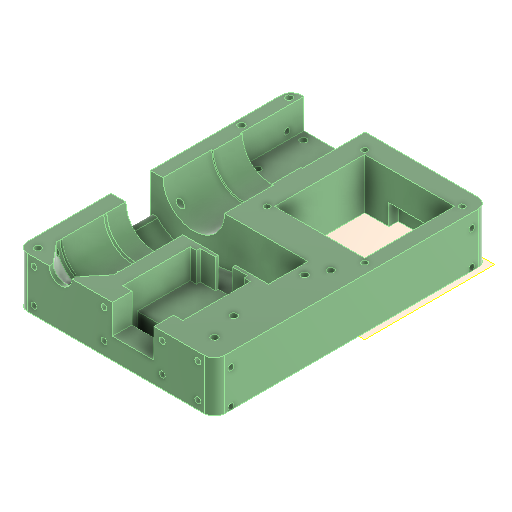
# Autodesk Inventor part: 60_Planktoscope_Base_half1
Saved by Autodesk Inventor 2024.1 (Build 281209000, 209)
## iProperties
Created: 2024-03-03
Part Number: 60_Planktoscope_Base_half1
Material: Generisch
Document SubType Name: Modeling
Designer: diederichbenedict
Density: 1 g/cm^3
Appearance: Glatt - Waldgrün
Author: diederichbenedict
Autodesk Inventor part; units mm, degrees
ref_plane "YZ Plane" through (0, 0, 0) normal (1, 0, 0) x (0, 1, 0)
ref_plane "XZ Plane" through (0, 0, 0) normal (0, 1, 0) x (-1, 0, 0)
ref_plane "Arbeitsebene1" through (0, 0, 0) normal (0, 0, 1) x (1, 0, 0)
ref_plane "Arbeitsebene2" through (-59.4, -108.46, 24.3) normal (0, 0, -1) x (0, 1, 0)
sketch "Skizze1" plane through (0, 0, 0) normal (0, 0, 1) x (1, 0, 0)
  line L0 (-24.5, 28.5) -> (24.5, 28.5) construction
  arc A0 (-24.5, 28.5) -> (-28.5, 24.5) centre (-24.5, 24.5) ccw construction
  line L1 (-28.5, -24.5) -> (-28.5, 24.5) construction
  arc A1 (-28.5, -24.5) -> (-24.5, -28.5) centre (-24.5, -24.5) ccw construction
  line L2 (24.5, -28.5) -> (-24.5, -28.5) construction
  arc A2 (24.5, -28.5) -> (28.5, -24.5) centre (24.5, -24.5) ccw construction
  line L3 (28.5, 24.5) -> (28.5, -24.5) construction
  arc A3 (28.5, 24.5) -> (24.5, 28.5) centre (24.5, 24.5) ccw construction
  circle A4 centre (15.5, -15.5) radius 2 construction
  circle A5 centre (-15.5, -15.5) radius 2 construction
  circle A6 centre (-15.5, 15.5) radius 2 construction
  circle A7 centre (15.5, 15.5) radius 2 construction
  circle A8 centre (0, 0) radius 11.5 construction
  circle A9 centre (23.5, -23.5) radius 2 construction
  circle A10 centre (-23.5, -23.5) radius 2 construction
  circle A11 centre (-23.5, 23.5) radius 2 construction
  circle A12 centre (23.5, 23.5) radius 2 construction
  line L4 (21.15, 14.15) -> (21.15, -14.15) construction
  line L5 (14.15, 21.15) -> (21.15, 14.15) construction
  line L6 (-14.15, 21.15) -> (14.15, 21.15) construction
  line L7 (-21.15, 14.15) -> (-14.15, 21.15) construction
  line L8 (-21.15, -14.15) -> (-21.15, 14.15) construction
  line L9 (-14.15, -21.15) -> (-21.15, -14.15) construction
  line L10 (14.15, -21.15) -> (-14.15, -21.15) construction
  line L11 (21.15, -14.15) -> (14.15, -21.15) construction
  line L12 (17.15, 21.15) -> (14.15, 21.15) construction
  line L13 (21.15, 14.15) -> (14.15, 21.15) construction
  line L14 (21.15, 14.15) -> (21.15, 17.15) construction
  line L15 (21.15, 17.15) -> (17.15, 21.15) construction
  line L16 (21.1433, 21.15) -> (-21.15, 21.15) construction
  line L17 (-21.15, 21.15) -> (-21.15, -21.15) construction
  line L18 (-21.15, -21.15) -> (21.1433, -21.15) construction
  line L19 (21.1433, -21.15) -> (21.1433, 21.15) construction
  line L20 (21.6433, 21.65) -> (-21.65, 21.65)
  line L21 (-21.65, 21.65) -> (-21.65, -21.65)
  line L22 (-21.65, -21.65) -> (21.6433, -21.65)
  line L23 (21.6433, -21.65) -> (21.6433, 21.65)
  circle A13 centre (23.5, 23.5) radius 1.4
  circle A14 centre (23.5, -23.5) radius 1.4
  circle A15 centre (-23.5, 23.5) radius 1.4
  circle A16 centre (-23.5, -23.5) radius 1.4
  line L24 (-58.0629, 31.15) -> (-46.7147, 31.15) construction
  line L25 (-24.5, 28.5) -> (24.5, 28.5) construction
  line L26 (-58.15, -108.944) -> (-33.15, -108.944) construction
  line L27 (-60.15, 4.6456) -> (-60.15, 29.65) construction
  line L28 (28.5, 31.15) -> (-66.5, 31.15) construction
  line L29 (-66.5, 31.15) -> (-66.5, -100.85) construction
  line L30 (-66.5, -100.85) -> (28.5, -100.85) construction
  line L31 (28.5, -100.85) -> (28.5, 31.15) construction
  line L32 (28.5, 31.15) -> (-66.5, 31.15)
  line L33 (-66.5, 31.15) -> (-66.5, -100.85)
  line L34 (-66.5, -100.85) -> (28.5, -100.85)
  line L35 (28.5, -100.85) -> (28.5, 31.15)
  circle A17 centre (-34.65, 27.15) radius 1.6 projected
  circle A18 centre (-35.65, 4.15) radius 1.55 projected
  arc A19 (-35.0696, 29.65) -> (-37.5716, 27.1718) centre (-35.0717, 27.15) ccw construction
  line L36 (-32.3578, 29.6503) -> (-35.0696, 29.6501) construction
  line L37 (-32.3578, 29.6503) -> (-32.3574, 2.149) construction
  spline S0 degree 3 poles (-33.2494, 1.4648) (-33.1945, 1.4704) (-33.1402, 1.4798) (-33.0852, 1.4932) (-33.0302, 1.5066) (-32.9745, 1.5241) (-32.9218, 1.5443) (-32.869, 1.5646) (-32.8192, 1.5877) (-32.7741, 1.6117) (-32.729, 1.6358) (-32.6887, 1.6608) (-32.6523, 1.6864) (-32.6158, 1.712) (-32.5833, 1.7382) (-32.5542, 1.7648) (-32.5251, 1.7914) (-32.4996, 1.8183) (-32.4775, 1.8453) (-32.4554, 1.8722) (-32.4367, 1.899) (-32.4213, 1.9255) (-32.4059, 1.952) (-32.3937, 1.978) (-32.3842, 2.0033) (-32.3747, 2.0286) (-32.3679, 2.0532) (-32.3636, 2.0778) (-32.3593, 2.1023) (-32.3574, 2.1268) (-32.3574, 2.149) knots 0 0 0 0 0.1 0.1 0.1 0.2 0.2 0.2 0.3 0.3 0.3 0.4 0.4 0.4 0.5 0.5 0.5 0.6 0.6 0.6 0.7 0.7 0.7 0.8 0.8 0.8 0.9 0.9 0.9 1 1 1 1 construction
  spline S1 degree 3 poles (-58.0506, 1.4648) (-57.9483, 1.4544) (-57.7309, 1.4485) (-57.3891, 1.4505) (-57.0142, 1.4499) (-56.6055, 1.45) (-56.1597, 1.45) (-55.6728, 1.45) (-55.1399, 1.45) (-54.5557, 1.45) (-53.9136, 1.45) (-53.2059, 1.45) (-52.4235, 1.45) (-51.5547, 1.45) (-50.5859, 1.45) (-49.498, 1.45) (-48.2725, 1.45) (-46.9373, 1.45) (-45.5731, 1.45) (-44.2623, 1.45) (-43.0442, 1.45) (-41.9119, 1.45) (-40.8595, 1.45) (-39.8813, 1.45) (-38.9722, 1.45) (-38.1274, 1.45) (-37.3425, 1.45) (-36.6135, 1.45) (-35.9369, 1.45) (-35.3097, 1.45) (-34.7295, 1.45) (-34.1949, 1.45) (-33.7068, 1.4499) (-33.3956, 1.4501) (-33.2494, 1.4648) knots 0 0 0 0 0.012454 0.026265 0.041356 0.057789 0.075708 0.095278 0.116688 0.140158 0.165945 0.194355 0.225757 0.26059 0.299437 0.342945 0.392182 0.44767 0.504448 0.55719 0.606219 0.651791 0.694148 0.733518 0.770107 0.804111 0.835704 0.865049 0.892289 0.917546 0.940917 0.962464 0.982201 1 1 1 1 construction
  spline S2 degree 3 poles (-58.9429, 2.1479) (-58.9428, 2.1323) (-58.9408, 2.1003) (-58.9319, 2.0518) (-58.9165, 2.0024) (-58.8947, 1.9528) (-58.866, 1.9029) (-58.8299, 1.8528) (-58.786, 1.8026) (-58.7333, 1.7522) (-58.6711, 1.7019) (-58.5978, 1.6519) (-58.512, 1.6028) (-58.4118, 1.556) (-58.2981, 1.5143) (-58.1761, 1.4822) (-58.092, 1.469) (-58.0506, 1.4648) knots 0.000644 0.000644 0.000644 0.000644 0.046478 0.094952 0.144249 0.194804 0.247064 0.301535 0.358802 0.419552 0.484614 0.554981 0.631878 0.716385 0.809647 0.906987 1 1 1 1 construction
  line L38 (-58.9426, 2.1485) -> (-58.9422, 29.6503) construction
  line L39 (-58.9422, 29.6503) -> (-56.2298, 29.6501) construction
  arc A20 (-53.7284, 27.1718) -> (-56.2298, 29.65) centre (-56.2283, 27.15) ccw construction
  line L40 (-53.7228, 26.5387) -> (-53.7284, 27.1718) construction
  arc A21 (-53.7228, 26.5387) -> (-52.4229, 25.25) centre (-52.4229, 26.55) ccw construction
  line L41 (-38.8771, 25.25) -> (-52.4229, 25.25) construction
  arc A22 (-38.8771, 25.25) -> (-37.5772, 26.5387) centre (-38.8771, 26.55) ccw construction
  line L42 (-37.5772, 26.5387) -> (-37.5716, 27.1718) construction
  circle A23 centre (-56.65, 27.15) radius 1.6 projected
  line L43 (-58.35, 24.2) -> (-35.55, 24.2) construction
  line L44 (-58.35, 8.8) -> (-58.35, 24.2) construction
  line L45 (-32.95, 8.8) -> (-58.35, 8.8) construction
  line L46 (-32.95, 21.2) -> (-32.95, 8.8) construction
  line L47 (-35.55, 24.2) -> (-32.95, 21.2) construction
  circle A24 centre (-55.65, 4.15) radius 1.55 projected
  circle A25 centre (-51.65, 5.65) radius 1.1 construction
  circle A26 centre (-39.65, 5.65) radius 1.1 construction
  circle A27 centre (-35.65, 4.15) radius 1.55 construction
  circle A28 centre (-34.65, 27.15) radius 1.6 construction
  point P0 (0, 0)
  dimension "d0" = 0.5
  dimension "d1" = 2.8
  dimension "d2" = 2.8
  dimension "d3" = 2.8
  dimension "d4" = 2.8
  dimension "d5" = 95
  dimension "d6" = 132
  dimension "d41" = 31.15
  constraints: 32 end point, 8 parallel, 4 centre point, 4 coincident, 4 perpendicular, 3 horizontal, 3 other
  measures "d0" distance between parallel lines of L19 L23
  measures "d1" diameter of A13
  measures "d2" diameter of A14
  measures "d3" diameter of A15
  measures "d4" diameter of A16
  measures "d5" distance of L30.end L29.end
  measures "d6" distance of L29.end L28.end
  measures "d41" distance from line of L28 point (0, 0)
extrude "Extrusion1" add sketch "Skizze1" along normal up to surface (24.3 mm away)
sketch "Skizze2" plane through (-66.5, 31.15, 24.3) normal (0, 0, 1) x (1, 0, 0)
  line L0 (44.85, -9.5) -> (88.1433, -9.5) projected
  line L1 (88.1433, -9.5) -> (88.1433, -52.8) projected
  line L2 (88.1433, -52.8) -> (44.85, -52.8) projected
  line L3 (44.85, -52.8) -> (44.85, -9.5) projected
  circle A0 centre (90, -7.65) radius 1.4 projected
  circle A1 centre (90, -54.65) radius 1.4 projected
  circle A2 centre (43, -7.65) radius 1.4 projected
  circle A3 centre (43, -54.65) radius 1.4 projected
  circle A4 centre (31.85, -4) radius 1.6 projected
  circle A5 centre (30.85, -27) radius 1.55 projected
  circle A6 centre (9.85, -4) radius 1.6 projected
  circle A7 centre (10.85, -27) radius 1.55 projected
  line L4 (95, 0) -> (0, 0) projected
  line L5 (0, 0) -> (0, -132) projected
  line L6 (0, -132) -> (95, -132) projected
  line L7 (95, -132) -> (95, 0) projected
  line L8 (7.35, -118.91) -> (7.35, -120.06)
  arc A8 (7.35, -118.91) -> (7.35, -117.91) centre (7.35, -118.41) ccw construction
  line L9 (7.35, -96.06) -> (7.35, -117.91) construction
  line L10 (7.35, -85.56) -> (7.35, -94.56)
  line L11 (6.25, -85.56) -> (35.45, -85.56) projected
  line L12 (6.25, -70.56) -> (6.25, -85.56)
  line L13 (6.25, -44.56) -> (6.25, -70.06)
  line L14 (6.9535, -41.86) -> (6.8517, -30.1979)
  line L15 (33.2, -30.2) -> (33.2, -41.66)
  line L16 (6.9, -41.86) -> (6.9, -44.56)
  line L17 (6.25, -44.56) -> (35.45, -44.56) projected
  line L18 (20.85, -132) -> (20.85, 0) construction
  line L19 (15.35, -128.06) -> (15.35, -132)
  line L20 (7.35, -96.06) -> (7.35, -94.56)
  line L21 (7.35, -85.56) -> (6.25, -85.56)
  line L22 (6.25, -70.56) -> (6.25, -70.06)
  line L23 (15.1, -132) -> (15.1, -128.1636)
  line L24 (7.1, -120.1636) -> (7.1, -118.41)
  arc A9 (7.1, -118.41) -> (7.1, -118.41) centre (7.35, -118.41) ccw
  line L25 (7.1, -118.41) -> (7.1, -96.0507)
  line L26 (7.1, -96.0507) -> (7.1, -94.56)
  line L27 (7.1, -94.56) -> (7.1, -85.81)
  line L28 (7.1, -85.81) -> (6, -85.81)
  line L29 (6, -85.81) -> (6, -70.56)
  line L30 (6, -70.56) -> (6, -70.06)
  line L31 (6, -70.06) -> (6, -44.31)
  line L32 (6, -44.31) -> (35.45, -44.31)
  line L33 (6.8, -44.31) -> (6.8, -30.064)
  line L34 (6.8, -30.064) -> (20.85, -30.064)
  line L35 (20.85, -30.064) -> (20.85, -132)
  line L36 (15.1, -132) -> (20.85, -132)
  line L37 (7.1, -97.4127) -> (7.2407, -96.0654)
  line L38 (7.2407, -96.0654) -> (7.1, -96.0507)
  circle A10 centre (7.1, -117.9136) radius 0.5
  line L39 (7.35, -120.06) -> (15.35, -129.594) construction
  line L40 (15.35, -130.03) -> (7.1, -120.198)
  line L41 (7.1, -120.198) -> (7.1, -120.1636)
  point P0 (66.5, -31.15)
  point P1 (20.85, -85.56)
  point P2 (20.85, -44.56)
  point P3 (20.85, -44.31)
  point P4 (7.1, -118.4136)
  point P5 (7.1, -117.4136)
  point P6 (15.1, -129.7321)
  point P7 (6.9, -44.31)
  dimension "d9" = 0.25
  dimension "d74" = 1
  dimension "d75" = 2.25
  constraints: 64 end point, 11 vertical, 7 point on line, 5 perpendicular, 4 point on circle, 3 centre point, 2 collinear, 1 horizontal, 1 midpoint, 1 parallel, 30 other
  measures "d9" distance between parallel lines of L9 L25
  measures "d74" diameter of A10
  measures "d75" distance of A10.centre L24.start
revolve "Umdrehung1" cut sketch "Skizze2" angle 360 about axis through (-45.65, -100.85, 24.3) along (0, 1, 0) contours L6 L19 L40 L41 L24 A9 A10 L25 L37 L38 L26 L27 L28 L29 L30 L31 L32 L16 L17 L13 L22 L12 L11 L35 | L11 L12 L22 L13 L17 L35 | L17 L16 L32 L35 | L32 L33 L34 L35 | A10 A9
sketch "Skizze3" plane through (-66.5, 31.15, 24.3) normal (0, 0, 1) x (1, 0, 0)
  line L0 (41.8499, -119.66) -> (41.8499, -113.96) projected
  line L1 (69.8499, -119.66) -> (69.8499, -113.96) projected
  line L2 (47.9499, -122.06) -> (63.7499, -122.06) projected
  line L3 (44.8499, -88.76) -> (66.8499, -88.76) projected
  line L4 (44.8499, -90.56) -> (44.8499, -88.76)
  line L5 (66.8499, -90.56) -> (66.8499, -88.76)
  line L6 (41.8499, -122.06) -> (69.8499, -122.06)
  line L7 (69.8499, -122.06) -> (69.8499, -90.56)
  line L8 (69.8499, -90.56) -> (41.8499, -90.56)
  line L9 (41.8499, -90.56) -> (41.8499, -122.06)
  line L10 (65.8499, -140.6578) -> (45.8499, -140.6578)
  line L11 (45.8499, -140.6578) -> (45.8499, -122.06)
  line L12 (45.8499, -122.06) -> (65.8499, -122.06)
  line L13 (65.8499, -122.06) -> (65.8499, -140.6578)
  line L14 (65.8499, -140.6578) -> (45.8499, -122.06) construction
  line L15 (45.8499, -140.6578) -> (65.8499, -122.06) construction
  line L16 (41.3499, -122.56) -> (70.3499, -122.56)
  line L17 (70.3499, -122.56) -> (70.3499, -90.06)
  line L18 (70.3499, -90.06) -> (41.3499, -90.06)
  line L19 (41.3499, -90.06) -> (41.3499, -122.56)
  line L20 (67.3499, -90.56) -> (67.3499, -88.26)
  line L21 (67.3499, -88.26) -> (44.3499, -88.26)
  line L22 (44.3499, -88.26) -> (44.3499, -90.56)
  line L23 (60.0306, -74.6503) -> (51.6692, -74.6503)
  line L24 (51.6692, -74.6503) -> (51.6692, -88.26)
  line L25 (51.6692, -88.26) -> (60.0306, -88.26)
  line L26 (60.0306, -88.26) -> (60.0306, -74.6503)
  line L27 (60.0306, -74.6503) -> (51.6692, -88.26) construction
  line L28 (51.6692, -74.6503) -> (60.0306, -88.26) construction
  point P0 (66.5, -31.15)
  point P1 (55.8499, -131.3589)
  point P2 (55.8499, -81.4552)
  point P3 (44.3499, -90.06)
  point P4 (45.8499, -122.56)
  point P5 (65.8499, -122.56)
  point P6 (67.3499, -90.06)
  dimension "d11" = 20
  dimension "d12" = 0.5
  dimension "d13" = 0.5
  constraints: 50 end point, 8 parallel, 4 midpoint, 4 perpendicular, 3 horizontal, 2 point on line, 2 vertical, 7 other
  measures "d11" distance of L11.end L12.end
  measures "d12" distance between parallel lines of L9 L19
  measures "d13" distance between parallel lines of L3 L21
extrude "Extrusion2" cut sketch "Skizze3" against normal blind 14.1
sketch "Skizze4" plane through (-60.5, -54.66, 24.3) normal (0, 1, 0) x (1, 0, 0)
  arc A0 (14.7163, 14.1976) -> (0.6736, 0.7871) centre (14.85, 0) ccw projected
  circle A1 centre (49.8499, -0.1) radius 2.3 projected
  circle A2 centre (14.85, 0) radius 14.1983
  circle A3 centre (49.8499, -0.1) radius 6
  circle A4 centre (14.85, 0) radius 25.1983
  circle A5 centre (49.8499, -0.1) radius 20
  line L0 (18.6637, 24.908) -> (52.8768, 19.6696)
  line L1 (49.8499, -0.1) -> (14.85, 0)
  point P0 (60.5, 24.3)
  point P1 (40.0482, -0.072)
  point P2 (29.8499, -0.0429)
  point P3 (35.666, -14.2003)
  point P4 (35.7468, 14.0811)
  dimension "d16" = 12
  dimension "d17" = 11
  dimension "d18" = 14
  constraints: 4 end point, 2 centre point, 2 coincident, 1 concentric, 8 other
  measures "d16" diameter of A3
extrude "Extrusion3" cut sketch "Skizze4" along normal blind 18 and the other way blind 1 contours A2 A0 | A5 A4 | A5 A4 L1 | L1 A4 A5 | A1 | A3 | A5 A4 | A4 L0 A5
sketch "Skizze5" plane through (-66.5, 31.15, 24.3) normal (0, 0, 1) x (1, 0, 0)
  line L0 (60.0306, -86.81) -> (60.0306, -88.26) projected
  line L1 (60.0306, -88.26) -> (67.3499, -88.26) projected
  line L2 (67.3499, -88.26) -> (67.3499, -90.06) projected
  line L3 (67.3499, -90.06) -> (70.3499, -90.06) projected
  line L4 (70.3499, -90.06) -> (70.3499, -122.56) projected
  line L5 (70.3499, -122.56) -> (65.8499, -122.56) projected
  line L6 (65.8499, -122.56) -> (65.8499, -132) projected
  line L7 (65.8499, -132) -> (95, -132) projected
  line L8 (95, -132) -> (95, 0) projected
  line L9 (95, 0) -> (0, 0) projected
  line L10 (26.35, -132) -> (45.8499, -132) projected
  line L11 (44.85, -9.5) -> (88.1433, -9.5) projected
  line L12 (88.1433, -9.5) -> (88.1433, -52.8) projected
  line L13 (88.1433, -52.8) -> (44.85, -52.8) projected
  line L14 (44.85, -52.8) -> (44.85, -9.5) projected
  circle A0 centre (90, -7.65) radius 1.4 projected
  circle A1 centre (90, -54.65) radius 1.4 projected
  circle A2 centre (43, -7.65) radius 1.4 projected
  circle A3 centre (43, -54.65) radius 1.4 projected
  circle A4 centre (31.85, -4) radius 1.6 projected
  circle A5 centre (30.85, -27) radius 1.55 projected
  circle A6 centre (9.85, -4) radius 1.6 projected
  circle A7 centre (10.85, -27) radius 1.55 projected
  line L15 (35.35, -1.5) -> (35.35, -27) projected
  line L16 (6.35, -26.9997) -> (6.35, -1.5) projected
  line L17 (35.35, -30.064) -> (6.35, -30.064)
  line L18 (6.35, -30.064) -> (6.35, 0)
  line L19 (6.35, 0) -> (35.35, 0)
  line L20 (35.35, 0) -> (35.35, -30.064)
  line L21 (35.65, -30.364) -> (6.05, -30.364)
  line L22 (6.05, -30.364) -> (6.05, 0.3)
  line L23 (6.05, 0.3) -> (35.65, 0.3)
  line L24 (35.65, 0.3) -> (35.65, -30.364)
  line L25 (45.8499, -132) -> (45.8499, -122.56) projected
  line L26 (45.8499, -122.56) -> (41.3499, -122.56) projected
  line L27 (41.3499, -122.56) -> (41.3499, -90.06) projected
  line L28 (41.3499, -90.06) -> (44.3499, -90.06) projected
  line L29 (44.3499, -90.06) -> (44.3499, -88.26) projected
  line L30 (44.3499, -88.26) -> (51.6692, -88.26) projected
  line L31 (51.6692, -88.26) -> (51.6692, -86.81) projected
  line L32 (0, -86.81) -> (0, -132) projected
  line L33 (51.6692, -86.81) -> (34.6, -86.81) projected
  line L34 (34.6, -86.81) -> (34.6, -96.0507) projected
  line L35 (34.6, -96.0507) -> (34.4593, -96.0654) projected
  line L36 (34.4593, -96.0654) -> (34.6, -97.4127) projected
  line L37 (34.6, -97.4127) -> (34.6, -117.4136) projected
  arc A8 (34.6, -117.4136) -> (34.6, -118.4136) centre (34.6, -117.9136) ccw projected
  line L38 (34.6, -118.4136) -> (34.6, -120.198) projected
  line L39 (34.6, -120.198) -> (26.35, -130.03) projected
  line L40 (26.35, -130.03) -> (26.35, -132) projected
  line L41 (75.8496, -86.81) -> (60.0306, -86.81) projected
  line L42 (0, 0) -> (0, -67.81) projected
  line L43 (0, -67.81) -> (6, -67.81) projected
  line L44 (6, -67.81) -> (6, -44.31) projected
  line L45 (6, -44.31) -> (6.8, -44.31) projected
  line L46 (6.8, -44.31) -> (6.8, -30.064) projected
  line L47 (6.8, -30.064) -> (34.9, -30.064) projected
  line L48 (34.9, -30.064) -> (34.9, -44.31) projected
  line L49 (34.9, -44.31) -> (35.7, -44.31) projected
  line L50 (35.7, -44.31) -> (35.7, -67.81) projected
  line L51 (35.7, -67.81) -> (75.8496, -67.81) projected
  line L52 (75.8496, -67.81) -> (75.8496, -86.81) projected
  line L53 (7.1, -86.81) -> (0, -86.81) projected
  line L54 (0, -132) -> (15.35, -132) projected
  line L55 (15.35, -132) -> (15.35, -130.03) projected
  line L56 (15.35, -130.03) -> (7.1, -120.198) projected
  line L57 (7.1, -120.198) -> (7.1, -118.4136) projected
  arc A9 (7.1, -118.4136) -> (7.1, -117.4136) centre (7.1, -117.9136) ccw projected
  line L58 (7.1, -117.4136) -> (7.1, -97.4127) projected
  line L59 (7.1, -97.4127) -> (7.2407, -96.0654) projected
  line L60 (7.2407, -96.0654) -> (7.1, -96.0507) projected
  line L61 (7.1, -96.0507) -> (7.1, -86.81) projected
  point P0 (66.5, -31.15)
  dimension "d23" = 0.3
  constraints: 16 end point, 4 parallel, 2 perpendicular, 1 horizontal, 1 point on line, 3 other
  measures "d23" distance between parallel lines of L20 L24
extrude "Extrusion4" cut sketch "Skizze5" against normal blind 14.3 contours L48 L17 L20 L15 L9 L24 L21 | L21 L46 L17 L48 | L21 L22 L9 L18 L16 L17 L46 | L17 L18 L16 L9 L20 L15 | L9 L22 L23 L24 | A4 | A5 | A6 | A7
sketch "Skizze6" plane through (0, 0, 0) normal (0, 0, -1) x (-1, 0, 0)
  line L0 (66.5, 31.15) -> (66.5, -100.85) construction
  line L1 (-28.5, 31.15) -> (66.5, 31.15) construction
  line L2 (-28.5, -100.85) -> (-28.5, 31.15) construction
  line L3 (66.5, -100.85) -> (-28.5, -100.85) construction
  circle A0 centre (55.65, 4.15) radius 1.55 projected
  circle A1 centre (56.65, 27.15) radius 1.6 projected
  circle A2 centre (35.65, 4.15) radius 1.55 projected
  circle A3 centre (34.65, 27.15) radius 1.6 projected
  circle A4 centre (23.5, -23.5) radius 1.4 projected
  circle A5 centre (23.5, 23.5) radius 1.4 projected
  circle A6 centre (-23.5, -23.5) radius 1.4 projected
  circle A7 centre (-23.5, 23.5) radius 1.4 projected
  line L4 (-21.6433, 21.65) -> (-21.6433, -21.65) projected
  line L5 (21.65, 21.65) -> (-21.6433, 21.65) projected
  line L6 (21.65, -21.65) -> (21.65, 21.65) projected
  line L7 (-21.6433, -21.65) -> (21.65, -21.65) projected
  line L8 (-18.5, -90.85) -> (-18.5, 21.15) construction
  line L9 (-18.5, 21.15) -> (56.5, 21.15) construction
  line L10 (56.5, 21.15) -> (56.5, -90.85) construction
  line L11 (56.5, -90.85) -> (-18.5, -90.85) construction
  point P0 (0, 0)
  point P1 (-18.5, -34.85)
  point P2 (-14.0855, -43.0199)
  point P3 (-14.0855, -77.1359)
  point P4 (63.5, 27.15)
  point P5 (63.5, 4.15)
  point P6 (61.2633, -96.1146)
  dimension "d26" = 10
  dimension "d34" = 3
  dimension "d35" = 3
  constraints: 8 end point, 2 coincident, 1 midpoint, 3 other
  measures "d26" distance between parallel lines of L3 L11
  measures "d34" distance from line of point (63.5, 4.15) L0
  measures "d35" distance from line of L0 point (63.5, 27.15)
hole "Bohrung1" at (18.5, -90.85, 0) at (18.5, -34.85, 0) at (14.0855, -43.0199, 0) at (14.0855, -77.1359, 0) at (-63.5, 4.15, 0) at (-63.5, 27.15, 0) at (-61.2633, -96.1146, 0) direction (0, 0, 1) diameter 3.3 end through all
sketch "Skizze8" plane through (-45.65, -100.85, 24.3) normal (0, -1, 0) x (1, 0, 0)
  line L0 (44.9999, 0) -> (74.15, 0) projected
  line L1 (44.9999, 0) -> (44.9999, -14.1) projected
  line L2 (44.9999, -14.1) -> (24.9999, -14.1) projected
  line L3 (24.9999, -14.1) -> (24.9999, 0) projected
  line L4 (5.5, 0) -> (24.9999, 0) projected
  line L5 (-20.85, -24.3) -> (74.15, -24.3) projected
  line L6 (66.15, -20.3) -> (66.15, -4) construction
  line L7 (66.15, -4) -> (48.9999, -4) construction
  line L8 (48.9999, -4) -> (48.9999, -18.1) construction
  line L9 (48.9999, -18.1) -> (20.9999, -18.1) construction
  line L10 (20.9999, -18.1) -> (20.9999, -4) construction
  line L11 (20.9999, -4) -> (8.8917, -4) construction
  arc A0 (-8.8917, -4) -> (8.8917, -4) centre (0, 0) ccw construction
  line L12 (-8.8917, -4) -> (-12.85, -4) construction
  line L13 (-12.85, -4) -> (-12.85, -20.3) construction
  line L14 (-12.85, -20.3) -> (66.15, -20.3) construction
  arc A1 (-5.5, 0) -> (5.5, 0) centre (0, 0) ccw projected
  line L15 (-20.85, 0) -> (-5.5, 0) projected
  line L16 (-20.85, -24.3) -> (-20.85, 0) projected
  line L17 (74.15, -24.3) -> (74.15, 0) projected
  point P0 (45.65, -24.3)
  constraints: 18 end point, 8 coincident, 2 point on circle, 1 centre point, 4 other
hole "Bohrung2" at (20.5, -100.85, 4) at (20.5, -100.85, 20.3) at (3.3499, -100.85, 6.2) at (-24.6501, -100.85, 6.2) at (-24.6501, -100.85, 20.3) at (-58.5, -100.85, 20.3) at (3.3499, -100.85, 20.3) at (-58.5, -100.85, 4) direction (0, 1, 0) diameter 2.8 depth 12 tip angle 118
sketch "Skizze10" plane through (-66.5, -55.66, 10.1497) normal (-1, 0, 0) x (0, 0, 1)
  line L0 (-10.1497, 86.81) -> (-10.1497, -45.19) projected
  line L1 (14.1503, 86.81) -> (14.1503, 19) projected
  line L2 (-12.6816, -37.19) -> (-12.6816, 54.56) construction
  line L3 (-12.6816, 54.56) -> (-4.6816, 54.56) construction
  line L4 (-4.6816, 54.56) -> (-4.6816, 65.06) construction
  line L5 (-4.6816, 65.06) -> (-12.6816, 65.06) construction
  line L6 (-12.6816, 65.06) -> (-12.6816, 77.56) construction
  line L7 (-12.6816, 77.56) -> (-4.6816, 77.56) construction
  line L8 (-4.6816, 77.56) -> (-4.6816, 78.81) construction
  line L9 (-4.6816, 78.81) -> (3.6184, 78.81) construction
  line L10 (3.6184, 78.81) -> (3.6184, 23) construction
  line L11 (3.6184, 23) -> (-4, 23) construction
  line L12 (-4, 23) -> (-4, -4) construction
  line L13 (-4, -4) -> (3.6184, -4) construction
  line L14 (3.6184, -4) -> (3.6184, -37.19) construction
  line L15 (3.6184, -37.19) -> (-12.6816, -37.19) construction
  line L16 (14.1503, 0) -> (0, 0) projected
  line L17 (0, 0) -> (0, 19) projected
  line L18 (0, 19) -> (14.1503, 19) projected
  line L19 (14.1503, 0) -> (14.1503, -45.19) projected
  line L20 (-10.1497, -45.19) -> (14.1503, -45.19) projected
  line L21 (-10.1497, 86.81) -> (14.1503, 86.81) projected
  point P0 (-10.1497, 55.66)
  constraints: 28 end point, 6 coincident
hole "Bohrung4" at (-66.5, -92.85, 13.7682) at (-66.5, -92.85, -2.5318) at (-66.5, -1.1, -2.5318) at (-66.5, -32.66, 13.7682) at (-66.5, 23.15, 13.7682) at (-66.5, 21.9, -2.5318) direction (1, 0, 0) diameter 2.8 depth 12 tip angle 118
fillet "Rundung1" radius 2 1 edges at (-66.5, -46.16, 10.1497)
sketch "Skizze12" plane through (-66.5, 31.15, 10.2) normal (0, 0, 1) x (1, 0, 0)
  line L0 (60.0306, -86.81) -> (51.6692, -86.81) projected
  line L1 (51.6692, -88.26) -> (51.6692, -86.81) projected
  line L2 (44.3499, -88.26) -> (51.6692, -88.26) projected
  line L3 (44.3499, -90.06) -> (44.3499, -88.26) projected
  line L4 (41.3499, -90.06) -> (44.3499, -90.06) projected
  line L5 (41.3499, -122.56) -> (41.3499, -90.06) projected
  line L6 (45.8499, -122.56) -> (41.3499, -122.56) projected
  line L7 (45.8499, -132) -> (45.8499, -122.56) projected
  line L8 (65.8499, -132) -> (45.8499, -132) projected
  line L9 (65.8499, -122.56) -> (65.8499, -132) projected
  line L10 (70.3499, -122.56) -> (65.8499, -122.56) projected
  line L11 (70.3499, -90.06) -> (70.3499, -122.56) projected
  line L12 (67.3499, -90.06) -> (70.3499, -90.06) projected
  line L13 (67.3499, -88.26) -> (67.3499, -90.06) projected
  line L14 (60.0306, -88.26) -> (67.3499, -88.26) projected
  line L15 (60.0306, -86.81) -> (60.0306, -88.26) projected
  line L16 (70.3499, -90.06) -> (70.3499, -122.56) projected
  line L17 (41.3499, -122.56) -> (70.3499, -122.56)
  line L18 (70.3499, -122.56) -> (70.3499, -115.56)
  line L19 (70.3499, -115.56) -> (41.3499, -115.56)
  line L20 (41.3499, -115.56) -> (41.3499, -122.56)
  point P0 (66.5, -31.15)
  dimension "d77" = 7
  constraints: 8 end point, 2 parallel, 1 horizontal, 1 perpendicular, 1 point on line
  measures "d77" distance of L18.end L17.end
extrude "Extrusion6" cut sketch "Skizze12" against normal through all contours L11 L10 L17 L6 L5 L19
sketch "Skizze13" plane through (0, 0, 0) normal (0, 0, -1) x (-1, 0, 0)
  line L0 (25.1501, -91.41) -> (-3.8499, -91.41) projected
  line L1 (-3.8499, -91.41) -> (-3.8499, -84.41) projected
  line L2 (-3.8499, -84.41) -> (25.1501, -84.41) projected
  line L3 (25.1501, -84.41) -> (25.1501, -91.41) projected
  line L4 (-21.6433, 21.65) -> (-21.6433, -21.65) projected
  line L5 (21.65, 21.65) -> (-21.6433, 21.65) projected
  line L6 (21.65, -21.65) -> (21.65, 21.65) projected
  line L7 (-21.6433, -21.65) -> (21.65, -21.65) projected
  circle A0 centre (-23.5, 23.5) radius 1.4 projected
  circle A1 centre (-23.5, -23.5) radius 1.4 projected
  circle A2 centre (23.5, 23.5) radius 1.4 projected
  circle A3 centre (23.5, -23.5) radius 1.4 projected
  circle A4 centre (34.65, 27.15) radius 1.6 projected
  circle A5 centre (35.65, 4.15) radius 1.55 projected
  circle A6 centre (56.65, 27.15) radius 1.6 projected
  circle A7 centre (55.65, 4.15) radius 1.55 projected
  line L8 (-28.5, -100.85) -> (-28.5, 31.15) projected
  line L9 (66.5, -100.85) -> (-28.5, -100.85) projected
  line L10 (66.5, 31.15) -> (66.5, -100.85) projected
  line L11 (-28.5, 31.15) -> (66.5, 31.15) projected
  line L12 (10.0034, 17.15) -> (-9.9966, 17.15)
  line L13 (-9.9966, 17.15) -> (-9.9966, 26.15)
  line L14 (-9.9966, 26.15) -> (10.0034, 26.15)
  line L15 (10.0034, 26.15) -> (10.0034, 17.15)
  line L16 (10.0034, 17.15) -> (-9.9966, 26.15) construction
  line L17 (-9.9966, 17.15) -> (10.0034, 26.15) construction
  point P0 (0, 0)
  point P1 (0.0034, 21.65)
  dimension "d80" = 20
  dimension "d81" = 9
  constraints: 12 end point, 3 midpoint, 2 parallel, 1 horizontal, 1 perpendicular
  measures "d80" distance of L13.end L14.end
  measures "d81" distance of L12.end L13.end
extrude "Extrusion7" cut sketch "Skizze13" against normal blind 10 contours L13 L14 L15 L5 | L5 L15 L12 L13
fillet "Rundung2" radius 5 4 edges at (28.5, -100.85, 12.15) (-66.5, -100.85, 12.15) (-66.5, 31.15, 12.15) (28.5, 31.15, 12.15)
sketch "Skizze14" plane through (28.5, -95.85, 0) normal (1, 0, 0) x (0, 0, -1)
  line L0 (9.752, 127) -> (9.752, -10) projected
  line L1 (9.752, -10) -> (-53.248, -10) projected
  line L2 (-53.248, -10) -> (-53.248, 127) projected
  line L3 (-53.248, 127) -> (9.752, 127) projected
  circle A0 centre (-25.748, 3) radius 1.4 projected
  circle A1 centre (-42.048, 119) radius 1.4 projected
  circle A2 centre (-25.748, 119) radius 1.4 projected
  circle A3 centre (-1.448, 3) radius 1.4 projected
  circle A4 centre (-17.748, 3) radius 1.4 projected
  circle A5 centre (-1.448, 119) radius 1.4 projected
  circle A6 centre (-17.748, 119) radius 1.4 projected
  circle A7 centre (-42.048, 3) radius 1.4 projected
  point P0 (0, 95.85)
  constraints: 4 coincident
hole "Bohrung6" at (28.5, 23.15, 1.448) at (28.5, 23.15, 17.748) at (28.5, -92.85, 1.448) at (28.5, -92.85, 17.748) direction (-1, 0, 0) diameter 2.8 depth 12 tip angle 118
